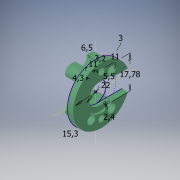
# Autodesk Inventor part: AS5047DEnclosureV2
Saved by Autodesk Inventor 2019.1 (Build 231200000, 200)
## iProperties
Created: 2018-06-30
Part Number: AS5047DEnclosureV2
Material: Generisch
Document SubType Name: Modeling
Designer: JochenAlt
Density: 1 g/cm^3
Appearance: Glatt - dunkelseegrün
Author: JochenAlt
Autodesk Inventor part; units mm, degrees
ref_plane "YZ Plane" through (0, 0, 0) normal (1, 0, 0) x (0, 1, 0)
ref_plane "XZ Plane" through (0, 0, 0) normal (0, 1, 0) x (-1, 0, 0)
ref_plane "Arbeitsebene1" through (0, 0, 0) normal (1, 0, 0) x (0, 0, -1)
sketch "Skizze1" plane through (0, 0, 0) normal (1, 0, 0) x (0, 0, -1)
  circle A0 centre (0, 0) radius 5.5
  line L0 (-24.52, 0) -> (24.52, 0) construction
  line L1 (0, -23.5528) -> (0, 22.3555) construction
  line L2 (8.89, -5.5) -> (-8.89, -5.5) construction
  line L3 (-8.89, -5.5) -> (-8.89, 5.5) construction
  line L4 (-8.89, 5.5) -> (8.89, 5.5) construction
  line L5 (8.89, 5.5) -> (8.89, -5.5) construction
  circle A1 centre (8.89, 5.5) radius 1.2
  circle A2 centre (-8.89, 5.5) radius 1.2
  arc A3 (-15.3, 0) -> (14.8761, 3.5767) centre (0, 0) ccw
  arc A4 (4.4, 3.3) -> (-4.4, 3.3) centre (0, 0) ccw
  circle A5 centre (8.89, -5.5) radius 1.2
  circle A6 centre (-8.89, -5.5) radius 1.2
  line L6 (-5.89, -5.5) -> (-5.89, 5.5)
  arc A7 (-5.89, 5.5) -> (-11.89, 5.5) centre (-8.89, 5.5) ccw
  arc A8 (11.89, 5.5) -> (5.89, 5.5) centre (8.89, 5.5) ccw
  line L7 (5.89, -5.5) -> (5.89, 5.5)
  circle A9 centre (8.89, -5.5) radius 2.15
  circle A10 centre (8.89, 5.5) radius 2.15
  circle A11 centre (-8.89, 5.5) radius 2.15
  circle A12 centre (0, 0) radius 11 construction
  circle A13 centre (-11, 0) radius 1.6
  circle A14 centre (11, 0) radius 1.6
  arc A15 (-11.89, -5.5) -> (-5.89, -5.5) centre (-8.89, -5.5) ccw
  arc A16 (5.89, -5.5) -> (11.89, -5.5) centre (8.89, -5.5) ccw
  line L8 (5.5, 0) -> (5.5, 14.2773)
  line L9 (-5.5, 0) -> (-5.5, 14.2773)
  arc A17 (15.3, 0) -> (5.5, 14.2773) centre (0, 0) ccw
  arc A18 (-5.5, 14.2773) -> (-15.3, 0) centre (0, 0) ccw
  line L10 (11.89, -5.5) -> (11.89, -3.1258)
  line L11 (11.89, 3.1258) -> (11.89, 5.5)
  line L12 (-11.89, -5.5) -> (-11.89, -3.1258)
  line L13 (-11.89, 3.1258) -> (-11.89, 5.5)
  circle A19 centre (11, 0) radius 3.25
  circle A20 centre (-11, 0) radius 3.25
  circle A21 centre (-8.89, -5.5) radius 2.15
  dimension "d2" = 11
  dimension "d19" = 11
  dimension "d20" = 17.78
  dimension "d22" = 2.4
  dimension "d29" = 15.3
  dimension "d30" = 5.5
  dimension "d38" = 3
  dimension "d52" = 22
  dimension "d53" = 3.2
  dimension "d55" = 6.5
  dimension "d60" = 4.3
  constraints: 26 point on circle, 24 end point, 22 centre point, 19 coincident, 14 tangent, 10 equal radius, 5 parallel, 2 point on line, 1 horizontal, 1 perpendicular, 3 other
  measures "d2" diameter of A0
  measures "d19" distance of L2.end L3.end
  measures "d20" distance of L3.end L4.end
  measures "d22" diameter of A1
  measures "d29" radius of A3
  measures "d30" radius of A4
  measures "d38" radius of A7
  measures "d52" diameter of A12
  measures "d53" diameter of A13
  measures "d55" diameter of A20
  measures "d60" diameter of A21
extrude "Extrusion7" add sketch "Skizze1" along normal blind 3.2 contours L8 A17 A3 A18 L9 A0 | A6 | A15 L12 A20 L13 A7 L6 | A20 | L11 A19 L10 A16 L7 A8 | A19 | A21
extrude "Extrusion3" add sketch "Skizze1" against normal blind 5 from surface at 0 contours A6 | A15 L12 A20 L13 A7 L6 | L11 A19 L10 A16 L7 A8 | A21
extrude "Extrusion4" add sketch "Skizze1" against normal blind 3 from surface at -5 contours A15 L12 A20 L13 A7 L6 | L11 A19 L10 A16 L7 A8 | A9 | A10 | A11 | A21
sketch "Skizze2" plane through (3.2, 0, 0) normal (1, 0, 0) x (0, 0, -1)
  circle A0 centre (0, 0) radius 8.25
  dimension "d57" = 16.5
  constraints: 1 centre point, 1 coincident
  measures "d57" diameter of A0
extrude "Extrusion9" cut sketch "Skizze2" against normal blind 1.2
